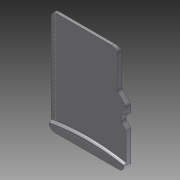
# Autodesk Inventor part: Part2
Saved by Autodesk Inventor 2011 (Build 150239000, 239)
## iProperties
Created: 2012-01-24
Part Number: Part2
Document SubType Name: Modeling
Designer: Seb Madgwick
Density: 1 g/cm^3
Author: Seb Madgwick
Autodesk Inventor part; units mm, degrees
ref_plane "YZ Plane" through (0, 0, 0) normal (1, 0, 0) x (0, 1, 0)
ref_plane "XZ Plane" through (0, 0, 0) normal (0, 1, 0) x (-1, 0, 0)
ref_plane "XY Plane" through (0, 0, 0) normal (0, 0, 1) x (1, 0, 0)
sketch "Sketch1" plane through (0, 0, 0) normal (0, 0, 1) x (1, 0, 0)
  line L0 (0, 0) -> (0, 15)
  line L1 (0, 15) -> (9.7, 15)
  line L2 (9.7, 15) -> (9.7, 9.5314)
  line L3 (9.7, 9.5314) -> (11, 8.2314)
  line L4 (11, 8.2314) -> (11, 7.1)
  line L5 (11, 7.1) -> (10.3, 7.1)
  line L6 (10.3, 7.1) -> (10.3, 5.9)
  line L7 (10.3, 5.9) -> (11, 5.2)
  line L8 (11, 5.2) -> (11, 0)
  line L9 (11, 0) -> (0, 0)
  dimension "d0" = 11
  dimension "d1" = 15
  dimension "d2" = 135
  dimension "d5" = 9.7
  dimension "d6" = 1.2
  dimension "d7" = 0.7
  dimension "d8" = 0.8
  dimension "d9" = 7.9
  dimension "d11" = 0
  constraints: 20 end point, 7 parallel, 1 perpendicular, 1 vertical
  measures "d0" distance of L8.end L0.start
  measures "d1" distance of L0.start L0.end
  measures "d2" angle of L3 L2
  measures "d5" distance of L0.end L1.end
  measures "d6" distance of L5.end L6.end
  measures "d7" distance between parallel lines of L4 L6
  measures "d8" distance from line of L4.end L3
  measures "d9" distance from line of L4.end L1
  measures "d11" distance between parallel lines of L4 L8
extrude "Extrusion1" add sketch "Sketch1" along normal blind 0.7
fillet "Fillet1" radius 0.8 4 edges at (9.7, 15, 0.35) (0, 15, 0.35) (0, 0, 0.35) (11, 0, 0.35)
fillet "Fillet2" radius 0.4 3 edges at (9.7, 9.5314, 0.35) (11, 8.2314, 0.35) (10.3, 5.9, 0.35)
fillet "Fillet3" radius 0.2 1 edges at (10.3, 7.1, 0.35)
sketch "Sketch3" plane through (0, 0.8, 0) normal (-1, 0, 0) x (0, 0, 1)
  line L0 (0, 0) -> (0, 13.4) projected
  line L1 (0, 14.2) -> (0.3, 14.2)
  line L2 (0.3, 14.2) -> (0, 13.68)
  line L3 (0, 14.2) -> (0, 13.68)
  line L4 (0.7, 14.2) -> (0, 14.2) projected
  point P0 (0, -0.8)
  dimension "d17" = 0.52
  dimension "d18" = 0
  dimension "d19" = 0.3
  constraints: 6 end point, 2 perpendicular, 1 point on line
  measures "d17" distance of L1.start L2.end
  measures "d18" distance between parallel lines of L4 L1
  measures "d19" distance of L1.start L1.end
extrude "Extrusion2" cut sketch "Sketch3" against normal through all
sketch "Sketch4" plane through (0, 0, 0.7) normal (0, 0, 1) x (1, 0, 0)
  line L0 (0, 0.8) -> (0, 14.2) projected
  arc A0 (0, 0.8) -> (0.8, 0) centre (0.8, 0.8) ccw projected
  line L1 (10.2, 0) -> (0.8, 0) projected
  arc A1 (10.2, 0) -> (11, 0.8) centre (10.2, 0.8) ccw projected
  line L2 (11, 5.2) -> (11, 0.8) projected
  arc A2 (11, 0.9915) -> (0, 0.9915) centre (5.5, -28.5) ccw
  point P0 (0, 0)
  dimension "d22" = 30
  dimension "d23" = 1.5
  dimension "d24" = 0.9915
  dimension "d25" = 0.9915
  constraints: 2 point on circle, 2 point on line, 1 centre point
  measures "d22" radius of A2
  measures "d23" distance edge to line of A2 L1
  measures "d24" distance from line of A2.end L1
  measures "d25" distance from line of A2.start L1
extrude "Extrusion3" add sketch "Sketch4" along normal blind 0.3
fillet "Fillet4" radius 0.2 2 edges at (5.5, 1.5, 0.7) (5.5, 1.5, 1)
equation "\"d24\" = d25"
body "Solid1"
